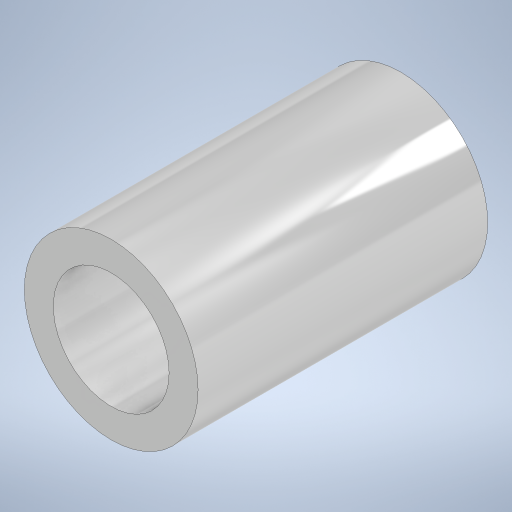
# Autodesk Inventor part: pi_spacer_10
Saved by Autodesk Inventor 2023 (Build 270158000, 158)
## iProperties
Created: 2023-06-18
Part Number: pi_spacer_10
Material: アルミニウム 6061-AHC
Document SubType Name: Modeling
Designer: blueh
Density: 2.7 g/cm^3
Appearance: アルミニウム - ダーク
Author: blueh
Autodesk Inventor part; units mm, degrees
ref_plane "YZ Plane" through (0, 0, 0) normal (1, 0, 0) x (0, 1, 0)
ref_plane "XZ Plane" through (0, 0, 0) normal (0, 1, 0) x (-1, 0, 0)
ref_plane "XY Plane" through (0, 0, 0) normal (0, 0, 1) x (1, 0, 0)
sketch "スケッチ1" plane through (0, 0, 0) normal (0, 0, 1) x (1, 0, 0)
  circle A0 centre (0, 0) radius 2
  circle A1 centre (0, 0) radius 3
  dimension "d0" = 4
  dimension "d1" = 6
  constraints: 2 centre point, 2 coincident
  measures "d0" diameter of A0
  measures "d1" diameter of A1
extrude "押し出し1" add sketch "スケッチ1" along normal mid plane 10
